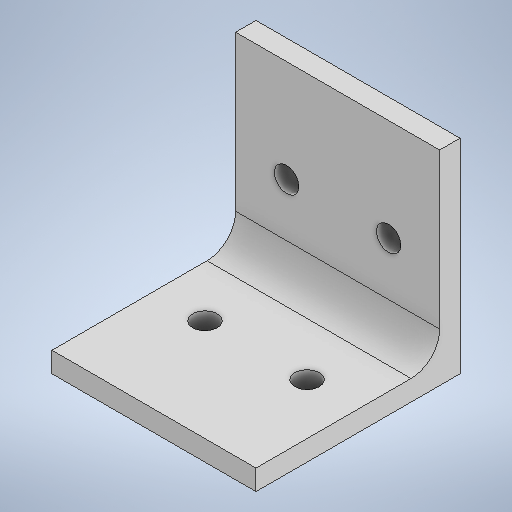
# Autodesk Inventor part: lclamp
Saved by Autodesk Inventor 2025.1 (Build 291241000, 241)
## iProperties
Created: 2025-11-11
Part Number: lclamp
Material: Generic
Document SubType Name: Modeling
Designer: mukund
Density: 1 g/cm^3
Appearance: Default
Author: mukund
Autodesk Inventor part; units mm, degrees
ref_plane "YZ Plane" through (0, 0, 0) normal (1, 0, 0) x (0, 1, 0)
ref_plane "XZ Plane" through (0, 0, 0) normal (0, 1, 0) x (-1, 0, 0)
ref_plane "XY Plane" through (0, 0, 0) normal (0, 0, 1) x (1, 0, 0)
sketch "Sketch1" plane through (0, 0, 0) normal (1, 0, 0) x (0, 1, 0)
  line L0 (0, 0) -> (5, 0)
  line L1 (5, 0) -> (5, 50)
  line L2 (5, 50) -> (0, 50)
  line L3 (0, 50) -> (0, 0)
  line L4 (0, 0) -> (50, 0)
  line L5 (50, 0) -> (50, 5)
  line L6 (50, 5) -> (0, 5)
  line L7 (0, 5) -> (0, 0)
  point P0 (5, 5)
  dimension "d0" = 5
  dimension "d1" = 50
  dimension "d2" = 50
  dimension "d3" = 5
  constraints: 16 end point, 4 parallel, 2 horizontal, 2 perpendicular
  measures "d0" distance of L2.end L1.end
  measures "d1" distance of L1.end L0.end
  measures "d2" distance of L6.end L5.end
  measures "d3" distance of L5.end L4.end
extrude "Extrusion1" add sketch "Sketch1" along normal mid plane 50
fillet "Fillet1" radius 7 1 edges at (0, 5, 5)
sketch "Sketch2" plane through (-25, 50, 5) normal (0, 0, 1) x (1, 0, 0)
  line L0 (0, 0) -> (0, -50) projected
  line L1 (0, 0) -> (0, -25)
  line L2 (12.5, -25) -> (37.5, -25)
  circle A0 centre (12.5, -25) radius 3
  circle A1 centre (37.5, -25) radius 3
  point P0 (25, -50)
  dimension "d7" = 25
  dimension "d8" = 6
  dimension "d9" = 6
  constraints: 4 end point, 2 centre point, 2 coincident, 1 horizontal, 1 midpoint
  measures "d7" distance of L2.start L2.end
  measures "d8" diameter of A0
  measures "d9" diameter of A1
sketch "Sketch3" plane through (-25, 5, 50) normal (0, 1, 0) x (1, 0, 0)
  line L0 (0, 50) -> (0, 0) projected
  line L1 (0, 0) -> (0, 25)
  line L2 (12.5, 25) -> (37.5, 25)
  circle A0 centre (12.5, 25) radius 3
  circle A1 centre (37.5, 25) radius 3
  point P0 (25, 50)
  dimension "d10" = 25
  dimension "d11" = 6
  dimension "d12" = 6
  constraints: 4 end point, 2 centre point, 2 coincident, 1 horizontal, 1 midpoint
  measures "d10" distance of L2.start L2.end
  measures "d11" diameter of A0
  measures "d12" diameter of A1
extrude "Extrusion2" cut sketch "Sketch2" against normal blind 50
extrude "Extrusion3" cut sketch "Sketch3" against normal blind 50
body "Solid1"
